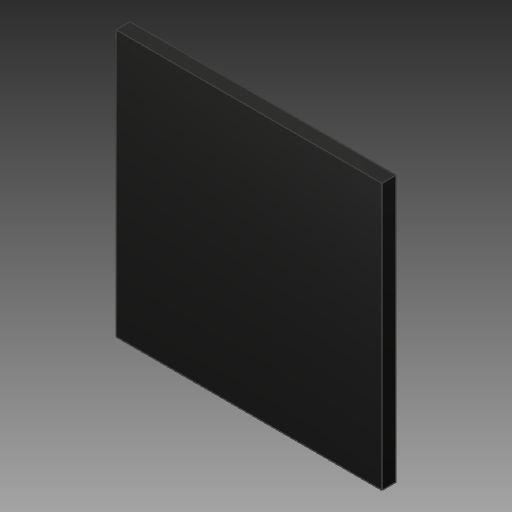
# Autodesk Inventor part: リング
Saved by Autodesk Inventor 2017 (Build 210142000, 142)
## iProperties
Part Number: リング
Material: 一般
Document SubType Name: Modeling
Designer: 雪村
Density: 1 g/cm^3
Appearance: 光沢 - 黒
Mass: 361000 g
Surface Area: 79800.3 cm^2
Volume: 361000 cm^3
Author: 雪村
Autodesk Inventor part; units mm, degrees
ref_plane "YZ Plane" through (0, 0, 0) normal (1, 0, 0) x (0, 1, 0)
ref_plane "XZ Plane" through (0, 0, 0) normal (0, 1, 0) x (-1, 0, 0)
ref_plane "XY Plane" through (0, 0, 0) normal (0, 0, 1) x (1, 0, 0)
sketch "スケッチ1" plane through (0, 0, 0) normal (0, 0, 1) x (1, 0, 0)
  line L0 (-950, -950) -> (-950, 950)
  line L1 (-950, 950) -> (950, 950)
  line L2 (950, 950) -> (950, -950)
  line L3 (950, -950) -> (-950, -950)
  point P0 (0, 0)
  point P1 (0, 0)
  dimension "d0" = 1900
  constraints: 8 end point, 1 coincident, 1 horizontal, 9 other
  measures "d0" distance of L0.end L1.end
extrude "押し出し1" add sketch "スケッチ1" along normal blind 100
sketch "スケッチ3" plane through (0, 0, 100) normal (0, 0, 1) x (1, 0, 0)
  circle A0 centre (0, 0) radius 0.005
  line L0 (-950, 950) -> (-950, -950) projected
  line L1 (-950, -950) -> (950, -950) projected
  line L2 (950, -950) -> (950, 950) projected
  line L3 (950, 950) -> (-950, 950) projected
  line L4 (-950, 950) -> (-950, 575)
  line L5 (-950, 950) -> (-950, -950) projected
  line L6 (-950, 575) -> (-575, 575)
  circle A1 centre (-575, 575) radius 0.005
  line L7 (950, -950) -> (950, -575)
  line L8 (950, -950) -> (950, 950) projected
  line L9 (950, -575) -> (575, -575)
  circle A2 centre (575, -575) radius 0.005
  line L10 (-950, -950) -> (0, -950)
  line L11 (0, -950) -> (0, -650)
  circle A3 centre (0, -650) radius 0.005
  line L12 (950, 950) -> (0, 950)
  line L13 (950, 950) -> (-950, 950) projected
  line L14 (0, 950) -> (0, 650)
  circle A4 centre (0, 650) radius 0.005
  line L15 (-950, -950) -> (-550, -950)
  line L16 (-950, -950) -> (950, -950) projected
  line L17 (-550, -950) -> (-550, -550)
  circle A5 centre (-550, -550) radius 0.005
  line L18 (950, 950) -> (550, 950)
  line L19 (550, 950) -> (550, 550)
  circle A6 centre (550, 550) radius 0.005
  line L20 (-950, -950) -> (-950, 0)
  line L21 (-950, 0) -> (-650, 0)
  line L22 (950, 950) -> (950, 0)
  line L23 (950, 0) -> (650, 0)
  circle A7 centre (-650, 0) radius 0.005
  circle A8 centre (650, 0) radius 0.005
  dimension "d8" = 0.01
  dimension "d9" = 375
  dimension "d10" = 375
  dimension "d11" = 0.01
  dimension "d12" = 375
  dimension "d13" = 375
  dimension "d14" = 0.01
  dimension "d15" = 300
  dimension "d16" = 0.01
  dimension "d17" = 300
  dimension "d18" = 0.01
  dimension "d19" = 400
  dimension "d20" = 400
  dimension "d21" = 0.01
  dimension "d22" = 400
  dimension "d23" = 400
  dimension "d24" = 0.01
  dimension "d25" = 300
  dimension "d26" = 300
  dimension "d27" = 0.01
  dimension "d28" = 0.01
  constraints: 32 end point, 9 centre point, 8 coincident, 5 point on line, 4 midpoint, 4 vertical, 3 horizontal
  measures "d8" diameter of A0
  measures "d9" distance of L0.start L4.end
  measures "d10" distance of L4.end L6.end
  measures "d11" diameter of A1
  measures "d12" distance of L1.end L7.end
  measures "d13" distance of L7.end L9.end
  measures "d14" diameter of A2
  measures "d15" distance of L10.end L11.end
  measures "d16" diameter of A3
  measures "d17" distance of L12.end L14.end
  measures "d18" diameter of A4
  measures "d19" distance of L0.end L15.end
  measures "d20" distance of L15.end L17.end
  measures "d21" diameter of A5
  measures "d22" distance of L2.end L18.end
  measures "d23" distance of L18.end L19.end
  measures "d24" diameter of A6
  measures "d25" distance of L20.end L21.end
  measures "d26" distance of L22.end L23.end
  measures "d27" diameter of A7
  measures "d28" diameter of A8
sketch "スケッチ3 outline for 押し出し2" plane through (0, 0, 100) normal (0, 0, 1) x (1, 0, 0)
  circle A0 centre (0, 0) radius 0.005
  circle A1 centre (-575, 575) radius 0.005
  circle A2 centre (575, -575) radius 0.005
  circle A3 centre (0, -650) radius 0.005
  circle A4 centre (0, 650) radius 0.005
  circle A5 centre (-550, -550) radius 0.005
  circle A6 centre (550, 550) radius 0.005
  circle A7 centre (-650, 0) radius 0.005
  circle A8 centre (650, 0) radius 0.005
extrude "押し出し2" cut sketch "スケッチ3 outline for 押し出し2" against normal blind 100
